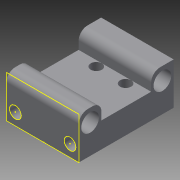
# Autodesk Inventor part: top
Saved by Autodesk Inventor 2014 (Build 180170000, 170)
## iProperties
Created: 2013-12-30
Part Number: top
Material: Generic
Document SubType Name: Modeling
Designer: stephen
Density: 1 g/cm^3
Appearance: Default
Author: stephen
Autodesk Inventor part; units mm, degrees
ref_plane "YZ Plane" through (0, 0, 0) normal (1, 0, 0) x (0, 1, 0)
ref_plane "XZ Plane" through (0, 0, 0) normal (0, 1, 0) x (-1, 0, 0)
ref_plane "XY Plane" through (0, 0, 0) normal (0, 0, 1) x (1, 0, 0)
sketch "Sketch1" plane through (0, 0, 0) normal (0, 1, 0) x (-1, 0, 0)
  line L0 (-16.4, 36.4) -> (17.6, 36.4)
  line L1 (17.6, 2.4) -> (-16.4, 2.4)
  line L2 (0, 36.4) -> (10, 36.4)
  line L3 (16.4, 6.0801) -> (17.6, 6.0801)
  line L4 (10, 24.9) -> (12.1364, 24.9)
  line L5 (-16.4, 2.4) -> (-16.4, 6.0801)
  line L6 (-16.4, 43.7199) -> (-16.4, 36.4)
  line L7 (17.6, 36.4) -> (17.6, 43.7199)
  line L8 (17.6, 6.0801) -> (17.6, 2.4)
  line L9 (0, 36.4) -> (0, 32.7199)
  line L10 (-16.4, 36.4) -> (17.6, 36.4)
  line L11 (17.6, 36.4) -> (17.6, 2.4)
  line L12 (17.6, 2.4) -> (-16.4, 2.4)
  line L13 (-16.4, 2.4) -> (-16.4, 36.4)
  circle A0 centre (-5.2589, 26.3219) radius 2
  line L14 (0, 19.4) -> (0, 2.4)
  circle A1 centre (5.2589, 26.3219) radius 2
  circle A2 centre (-5.2589, 12.4781) radius 2
  circle A3 centre (5.2589, 12.4781) radius 2
  point P0 (0, 0)
  point P1 (10, 2.4)
  point P2 (-10, 47.4)
  point P3 (-10, 2.4)
  point P4 (-17.6, 6.0801)
  point P5 (-17.6, 43.7199)
  point P6 (-10, 24.9)
  dimension "d1" = 34
  dimension "d4" = 10
  dimension "d5" = 4
  constraints: 30 end point, 8 parallel, 5 point on line, 4 centre point, 4 perpendicular, 2 horizontal, 2 symmetric about line, 1 collinear, 1 other
  measures "d1" distance between parallel lines of L1 L0
  measures "d4" distance of L2.start L2.end
  measures "d5" diameter of A0
extrude "Extrusion2" add sketch "Sketch1" along normal blind 9
sketch "Sketch7" plane through (-17.6, 0, 36.4) normal (0, 0, 1) x (1, 0, 0)
  line L0 (0, 0) -> (34, 0) projected
  line L1 (0, 9) -> (34, 9) projected
  line L2 (17, 9) -> (17, 0)
  line L3 (0, 9) -> (17, 9)
  circle A0 centre (30.6525, 4.2375) radius 2.0955
  circle A1 centre (7.2, 4.2375) radius 2.0955
  line L4 (18.8525, 9) -> (-33.0985, 9)
  line L5 (18.8525, 23.1318) -> (18.8525, -15.955)
  line L6 (0, 0) -> (0, 9) projected
  dimension "d16" = 4.7625
  dimension "d21" = 7.2
  constraints: 8 end point, 2 centre point, 2 midpoint, 1 collinear, 1 horizontal, 1 point on line
  measures "d16" distance from line of A1.centre L4
  measures "d21" distance from line of L6 A1.centre
extrude "Extrusion6" cut sketch "Sketch7" against normal up to next contours A1
sketch "Sketch8" plane through (-17.6, 0, 36.4) normal (0, 0, 1) x (1, 0, 0)
  circle A0 centre (7.2, 4.2375) radius 2.0955 projected
  line L0 (0, 9) -> (34, 9) projected
  line L1 (0, 0) -> (0, 9) projected
  line L2 (17, 9) -> (17, 4.5)
  circle A1 centre (7.2, 4.2375) radius 2.0955
  circle A2 centre (26.8, 4.2375) radius 2.0955
  line L3 (34, 0) -> (34, 9) projected
  point P0 (17.6, 0)
  dimension "d22" = 7.2
  dimension "d23" = 7.2
  dimension "d24" = 19.6
  constraints: 2 centre point, 2 end point, 1 coincident, 1 concentric, 1 midpoint, 1 parallel, 1 symmetric about line, 1 other
  measures "d22" distance from line of L3 A2.centre
  measures "d23" distance from line of L1 A0.centre
  measures "d24" distance of A2.centre A0.centre
extrude "Extrusion7" cut sketch "Sketch8" against normal up to next contours A2
sketch "Sketch10" plane through (16.4, 0, 2.4) normal (0, 0, -1) x (-1, 0, 0)
  line L0 (0, 0) -> (34, 0) projected
  line L1 (0, 9) -> (4, 9)
  line L2 (4, 9) -> (4, 0)
  line L3 (4, 0) -> (0, 0)
  line L4 (0, 0) -> (0, 9)
  point P0 (16.4, 0)
  dimension "d25" = 4
  constraints: 8 end point, 2 parallel, 1 horizontal, 1 perpendicular, 1 point on line
  measures "d25" distance of L2.end L3.end
extrude "Extrusion8" cut sketch "Sketch10" against normal through all
sketch "Sketch11" plane through (-17.6, 0, 2.4) normal (0, 0, -1) x (-1, 0, 0)
  line L0 (-30, 0) -> (0, 0) projected
  line L1 (0, 9) -> (-4, 9)
  line L2 (-4, 9) -> (-4, 0)
  line L3 (-4, 0) -> (0, 0)
  line L4 (0, 0) -> (0, 9)
  point P0 (-17.6, 0)
  dimension "d28" = 4
  constraints: 8 end point, 2 parallel, 1 horizontal, 1 perpendicular, 1 point on line
  measures "d28" distance of L3.end L2.end
extrude "Extrusion9" cut sketch "Sketch11" against normal through all
sketch "Sketch12" plane through (0, 9, 0) normal (0, 1, 0) x (1, 0, 0)
  line L0 (12.4, -36.4) -> (12.4, -2.4) projected
  line L1 (-13.6, -36.4) -> (12.4, -36.4)
  line L2 (12.4, -36.4) -> (12.4, -28.3219)
  line L3 (12.4, -28.3219) -> (-13.6, -28.3219)
  line L4 (-13.6, -28.3219) -> (-13.6, -36.4)
  point P0 (0, 0)
  constraints: 8 end point, 2 parallel, 1 horizontal, 1 perpendicular, 1 point on line
extrude "Extrusion10" add sketch "Sketch12" along normal blind 6
sketch "Sketch13" plane through (0, 9, 0) normal (0, 1, 0) x (1, 0, 0)
  line L0 (12.4, -28.3219) -> (12.4, -2.4) projected
  line L1 (-13.6, -2.4) -> (12.4, -2.4)
  line L2 (12.4, -2.4) -> (12.4, -10.4781)
  line L3 (12.4, -10.4781) -> (-13.6, -10.4781)
  line L4 (-13.6, -10.4781) -> (-13.6, -2.4)
  point P0 (0, 0)
  constraints: 8 end point, 2 parallel, 1 horizontal, 1 perpendicular, 1 point on line
extrude "Extrusion11" add sketch "Sketch13" along normal blind 6
sketch "Sketch14" plane through (12.4, 0, 36.4) normal (1, 0, 0) x (0, 0, -1)
  line L0 (0, 0) -> (0, 15) projected
  line L1 (8.0781, 9) -> (8.0781, 15) projected
  line L2 (0, 15) -> (8.0781, 15) projected
  line L3 (0, 0) -> (0, 6.35)
  line L4 (0, 6.35) -> (10.8068, 6.35)
  line L5 (4.039, 15) -> (4.039, 6.35)
  circle A0 centre (4.039, 10.389) radius 4.039
  circle A1 centre (4.039, 10.389) radius 3.175
  point P0 (36.4, 0)
  dimension "d35" = 6.35
  dimension "d36" = 6.35
  constraints: 6 end point, 3 tangent, 2 centre point, 2 perpendicular, 2 point on line, 1 coincident, 1 midpoint
  measures "d35" distance of L0.start L3.end
  measures "d36" diameter of A1
sketch "Sketch15" plane through (-13.6, 0, 36.4) normal (0, 0, 1) x (1, 0, 0)
  line L0 (0, 15) -> (0, 0) projected
  line L1 (0, 0) -> (26, 0) projected
  line L2 (26, 0) -> (26, 15) projected
  line L3 (0, 15) -> (26, 15) projected
  circle A0 centre (3.2, 4.2375) radius 2.0955 projected
  circle A1 centre (22.8, 4.2375) radius 2.0955 projected
  point P0 (13.6, 0)
extrude "Extrusion12" cut sketch "Sketch14" against normal up to next contours A1 L5 | L5 A1
sketch "Sketch16" plane through (12.4, 0, 36.4) normal (1, 0, 0) x (0, 0, -1)
  circle A0 centre (4.039, 10.389) radius 3.175 projected
  line L0 (34, 15) -> (34, 0) projected
  line L1 (25.9219, 15) -> (34, 15) projected
  line L2 (0, 15) -> (8.0781, 15) projected
  line L3 (4.039, 10.389) -> (34, 10.389)
  line L4 (29.961, 15) -> (29.961, 10.389)
  circle A1 centre (29.961, 10.389) radius 3.175
  point P0 (36.4, 0)
  dimension "d39" = 6.35
  constraints: 4 end point, 2 point on line, 1 centre point, 1 coincident, 1 midpoint, 1 parallel, 1 perpendicular
  measures "d39" diameter of A1
extrude "Extrusion13" cut sketch "Sketch16" against normal up to next contours A1 L3 | L3 L4 A1 | L4 L3 A1
fillet "Fillet1" radius 3.175 3 edges at (-0.6, 15, 28.3219) (-0.6, 15, 10.4781) (-0.6, 15, 36.4)
body "Solid2"
